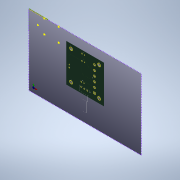
# Autodesk Inventor part: PCB_Temp
Saved by Autodesk Inventor 2021 (Build 250183000, 183)
## iProperties
Created: 2021-02-15
Part Number: PCB_Temp
Material: FR4
Document SubType Name: Modeling
Designer: James
Density: 1 g/cm^3
Appearance: Printed Circuit Board Green
Author: James
Autodesk Inventor part; units mm, degrees
ref_plane "YZ Plane" through (0, 0, 0) normal (1, 0, 0) x (0, 1, 0)
ref_plane "XZ Plane" through (0, 0, 0) normal (0, 1, 0) x (-1, 0, 0)
ref_plane "XY Plane" through (0, 0, 0) normal (0, 0, 1) x (1, 0, 0)
sketch "Sketch1" plane through (0, 0, 0) normal (0, 0, 1) x (1, 0, 0)
  line L0 (30, 30) -> (-30, 30)
  line L1 (-30, 30) -> (-30, -30)
  line L2 (-30, -30) -> (30, -30)
  line L3 (30, -30) -> (30, 30)
  line L4 (30, 30) -> (-30, -30) construction
  line L5 (-30, 30) -> (30, -30) construction
  circle A0 centre (20.4313, 28.5228) radius 1.5 projected
  circle A1 centre (66.4313, 28.5228) radius 1.5 projected
  circle A2 centre (66.4313, -15.9772) radius 1.5 projected
  circle A3 centre (20.4313, -15.9772) radius 1.5 projected
  circle A4 centre (20.4313, 28.5228) radius 1.5
  line L6 (-95.8555, 0) -> (165.4738, 0)
  line L7 (0, -104.3584) -> (0, 126.4825)
  line L8 (0, -104.3584) -> (0, 126.4825)
  line L9 (0, -104.3584) -> (0, 126.4825)
  circle A5 centre (-20.4313, 28.5228) radius 1.5
  circle A6 centre (-20.4313, 28.5228) radius 1.5
  circle A7 centre (20.4313, -28.5228) radius 1.5
  circle A8 centre (66.4313, -28.5228) radius 1.5
  point P0 (0, 0)
  dimension "width" = 60
  dimension "length" = 60
  constraints: 20 end point, 5 centre point, 4 symmetric about line, 3 vertical, 2 coincident, 2 horizontal, 2 midpoint, 2 parallel, 1 perpendicular, 12 other
  measures "width" distance of L2.end L1.end
  measures "length" distance of L1.end L0.end
extrude "Extrusion1" add sketch "Sketch1" along normal blind 1.6 contours L3 L6 L7 L0 A0 | A0 L0 | L3 L2 A7 L7 L6 | L7 L2 L1 L6 | L6 L1 L0 A5 L7 | L2 A7 | A5 L0 | A3 picked at (19.9626, 28.8581) picked at (19.7127, -28.0807) picked at (-20.9, 28.8581)
sketch "Sketch2" plane through (0, 0, 1.6) normal (0, 0, 1) x (1, 0, 0)
  circle A0 centre (20.4313, 28.5228) radius 1.5 projected
  circle A1 centre (66.4313, 28.5228) radius 1.5 projected
  circle A2 centre (66.4313, -15.9772) radius 1.5 projected
  circle A3 centre (20.4313, -15.9772) radius 1.5 projected
  line L0 (30, 30) -> (-30, 30) projected
  line L1 (-30, 30) -> (331.5267, 30) construction
  line L2 (331.5267, 30) -> (331.5267, -197.5417) construction
  line L3 (331.5267, -197.5417) -> (-30, -197.5417) construction
  line L4 (-30, -197.5417) -> (-30, 30) construction
  point P0 (0, 0)
  constraints: 2 other
body "Solid1"
